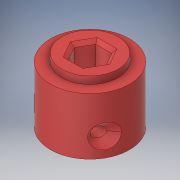
# Autodesk Inventor part: 2SidedSpoolV04
Saved by Autodesk Inventor 2019.3 (Build 233278000, 278)
## iProperties
Created: 2019-02-25
Part Number: 2SidedSpoolV04
Material: PC/ABS Plastic
Document SubType Name: Modeling
Designer: steele
Density: 0.357273 g/cm^3
Appearance: Smooth - Red
holeForString: 0.200 in
stringDiameter: 0.120 in
clearanceForString: 0.080 in
hexShaftDiameter: 0.500 in
clearanceForHexShaft: 0.023 in
hexDiameter: 0.523 in
supportChannels: 0.150 in
spoolInteriorDiameter: 1.500 in
spoolInteriroRadius: 0.750 in
spoolExteriorDiameter: 3.500 in
spoolExteriorRadius: 1.750 in
spoolFiletRadius: 0.075 in
holeCenter: 0.575 in
hexHoleChamfer: 0.063 in
stringHoleCenterFromHexShaft: 0.361 in
textCircleDiameter: 2.625 in
textHeight: 0.240 in
textDepth: 0.050 in
stringHoleChamfer: 0.125 in
spoolTotalHeight: 3.000 in
spaceHeight: 0.250 in
spacerDiameter: 0.950 in
spoolHeightWithoutSpacer: 2.750 in
Author: steele
Autodesk Inventor part; units mm, degrees
ref_plane "YZ Plane" through (0, 0, 0) normal (1, 0, 0) x (0, 1, 0)
ref_plane "XZ Plane" through (0, 0, 0) normal (0, 1, 0) x (-1, 0, 0)
sketch "Sketch9" plane through (0, 0, 0) normal (0, 1, 0) x (-1, 0, 0)
  circle A0 centre (0, 0) radius 19.05
  dimension "d53" = 38.1
  constraints: 1 centre point, 1 coincident
  measures "d53" diameter of A0
extrude "Extrusion6" add sketch "Sketch9" along normal mid plane 27.432
sketch "Sketch10" plane through (0, 13.716, 0) normal (0, 1, 0) x (1, 0, 0)
  circle A0 centre (0, 0) radius 13.589
  dimension "idWasher" = 27.178
  constraints: 1 centre point, 1 coincident
  measures "idWasher" diameter of A0
extrude "Extrusion7" add sketch "Sketch10" along normal blind 3.556
sketch "Sketch11" plane through (0, 17.272, 0) normal (0, 1, 0) x (1, 0, 0)
  line L0 (7.6623, 0) -> (3.8312, -6.6358)
  line L1 (3.8312, -6.6358) -> (-3.8312, -6.6358)
  line L2 (-3.8312, -6.6358) -> (-7.6623, 0)
  line L3 (-7.6623, 0) -> (-3.8312, 6.6357)
  line L4 (-3.8312, 6.6357) -> (3.8312, 6.6357)
  line L5 (3.8312, 6.6357) -> (7.6623, 0)
  point P0 (0, 0)
  point P1 (0, 0)
  dimension "d59" = 13.2715
  constraints: 12 end point, 1 coincident, 1 horizontal, 13 other
  measures "d59" distance between parallel lines of L1 L4
extrude "Extrusion8" cut sketch "Sketch11" against normal through all
sketch "Sketch12" plane through (0, 0, 0) normal (1, 0, 0) x (0, 1, 0)
  circle A0 centre (-4.572, 9.1758) radius 2.54
  line L0 (17.272, 0) -> (-13.716, 0) projected
  line L1 (-13.716, 19.05) -> (-13.716, -19.05) projected
  point P0 (0, 0)
  dimension "d62" = 5.08
  dimension "d63" = 9.1758
  dimension "oneThirdSpoolHeight" = 9.144
  constraints: 1 centre point
  measures "d62" diameter of A0
  measures "d63" distance from line of L0 A0.centre
  measures "oneThirdSpoolHeight" distance from line of A0.centre L1
extrude "Extrusion9" cut sketch "Sketch12" along normal through all both and the other way through all
chamfer "Chamfer5" distance 3.175 angle 45 2 edges at (16.6229, -7.1087, 9.3048) (-16.6229, -7.1087, 9.3048)
ref_plane "Work Plane2" through (0, 0, -19.05) normal (0, 0, 1) x (1, 0, 0)
sketch "Sketch13" plane through (0, 0, -19.05) normal (0, 0, 1) x (1, 0, 0)
  point P0 (0, 0)
  point P1 (0, 0)
  constraints: 1 coincident
hole "Hole2" at (0, 0, -19.05) direction (0, 0, 1) diameter 4.699 depth 12.4143 counterbore diameter 5.5372 counterbore depth 5.5626
chamfer "Chamfer6" distance 1.5875 angle 45 12 edges at (-5.7467, 17.272, -3.3179) (0, 17.272, -6.6357) (5.7467, 17.272, -3.3179) (5.7467, 17.272, 3.3179) (0, 17.272, 6.6358) (-5.7467, 17.272, 3.3179) (0, -13.716, 6.6358) (5.7467, -13.716, 3.3179) (5.7467, -13.716, -3.3179) (0, -13.716, -6.6357) (-5.7467, -13.716, -3.3179) (-5.7467, -13.716, 3.3179)
equation "\"d53\" = spoolInteriorDiameter"
equation "\"d59\" = hexDiameter"
equation "\"d62\" = holeForString"
equation "\"d63\" = stringHoleCenterFromHexShaft"
equation "\"oneThirdSpoolHeight\" = 0.333333 * singleSpoolHeight"
equation "\"d67\" = stringHoleChamfer"
equation "\"d77\" = hexHoleChamfer"
equation "\"holeForString\" = stringDiameter + clearanceForString"
equation "\"stringDiameter\" = 3.048"
equation "\"clearanceForString\" = 2.032"
equation "\"spoolHeightWithoutSpacer\" = 69.85"
equation "\"hexShaftDiameter\" = 12.7"
equation "\"clearanceForHexShaft\" = 0.5715"
equation "\"hexDiameter\" = hexShaftDiameter + clearanceForHexShaft"
equation "\"supportChannels\" = 3.81"
equation "\"spoolInteriorDiameter\" = 38.1"
equation "\"spoolInteriroRadius\" = 0.5 * spoolInteriorDiameter"
equation "\"spoolExteriorDiameter\" = 88.9"
equation "\"spoolExteriorRadius\" = 0.5 * spoolExteriorDiameter"
equation "\"spoolFiletRadius\" = 0.5 * supportChannels"
equation "\"holeCenter\" = 0.25 * spoolHeightWithoutSpacer - 0.75 * supportChannels"
equation "\"hexHoleChamfer\" = 1.5875"
equation "\"stringHoleCenterFromHexShaft\" = 0.5 * hexDiameter + 0.5 * holeForString"
equation "\"textCircleDiameter\" = 0.75 * spoolExteriorDiameter"
equation "\"textHeight\" = 6.096"
equation "\"textDepth\" = 1.27"
equation "\"stringHoleChamfer\" = 3.175"
equation "\"spoolTotalHeight\" = 76.2"
equation "\"spaceHeight\" = spoolTotalHeight - spoolHeightWithoutSpacer"
equation "\"spacerDiameter\" = 24.13"
equation "\"singleSpoolHeight\" = 27.432"
body "Solid1"
body "Solid2"
